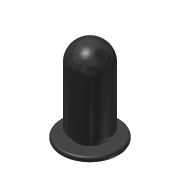
# Autodesk Inventor part: Bulb
Saved by Autodesk Inventor 2015 SP2 (Build 190223200, 223)
## iProperties
Created: 2016-12-12
Part Number: Bulb
Material: Rubber
Document SubType Name: Modeling
Designer: dsnyder
Density: 0.93 g/cm^3
Appearance: Rubber - Black - Version 1.1
Author: dsnyder
Autodesk Inventor part; units mm, degrees
ref_plane "YZ Plane" through (0, 0, 0) normal (1, 0, 0) x (0, 1, 0)
ref_plane "XZ Plane" through (0, 0, 0) normal (0, 1, 0) x (-1, 0, 0)
ref_plane "XY Plane" through (0, 0, 0) normal (0, 0, 1) x (1, 0, 0)
sketch "Sketch1" plane through (0, 0, 0) normal (0, 0, 1) x (1, 0, 0)
  line L0 (4.7625, 0) -> (6.35, 0)
  line L1 (6.35, 0) -> (6.35, 19.05)
  line L2 (0, 25.4) -> (0, 25.4)
  line L3 (0, 25.4) -> (0, 0)
  arc A0 (6.35, 19.05) -> (0, 25.4) centre (0, 19.05) ccw
  line L4 (4.7625, -1.5875) -> (9.525, -1.5875)
  line L5 (9.525, -1.5875) -> (9.525, -3.175)
  line L6 (9.525, -3.175) -> (0, -3.175)
  line L7 (0, -3.175) -> (0, -0.9465)
  line L8 (0, -0.9465) -> (0, 0)
  line L9 (4.7625, -1.5875) -> (4.7625, 0)
  point P0 (6.35, 25.4)
  dimension "d0" = 6.35
  dimension "d1" = 25.4
  dimension "d2" = 6.35
  dimension "d3" = 4.7625
  dimension "d4" = 1.5875
  dimension "d5" = 1.5875
  constraints: 20 end point, 4 parallel, 3 perpendicular, 2 horizontal, 2 point on circle, 2 point on line, 2 tangent, 1 centre point, 1 vertical
  measures "d0" distance of L2.end point (6.35, 25.4)
  measures "d1" distance between parallel lines of L0 L2
  measures "d2" radius of A0
  measures "d3" distance between parallel lines of L9 L8
  measures "d4" distance between parallel lines of L4 L0
  measures "d5" distance between parallel lines of L4 L6
revolve "Revolution1" add sketch "Sketch1" angle 360 about axis through (0, 25.4, 0) along (0, -1, 0)
shell "Shell1" thickness 1.5875 removed faces 1 at (0.831, -3.175, -0.7598)
fillet "Fillet1" radius 0.635 4 edges at (-6.35, 0, 0) (-9.525, -1.5875, 0) (-9.525, -3.175, 0) (-3.175, -3.175, 0.001)
body "Solid1"
